ring bowl (Autodesk Fusion 360 design; units mm, degrees)
Autodesk Fusion 360 part; units mm, degrees
note: some values were not read from the file. Set by a fixed rule: which sketch regions a step uses.
sketch "Sketch1" plane through (0, 0, 0) normal (0, 1, 0) x (1, 0, 0) in component "Component"
  circle A0 centre (0, 0) radius 70
  circle A1 centre (0, 0) radius 60
  dimension "d1" = 140
  dimension "d2" = 120
  constraint coincident A0.centre A1.centre
  measures "d1" diameter of A0
  measures "d2" diameter of A1
extrude "Extrude1" add sketch "Sketch1" along normal blind 10 in component "Component"
sketch "Sketch2" plane through (0, 0, 0) normal (0, -1, 0) x (1, 0, 0) in component "Component"
  circle A0 centre (0, 0) radius 60
  circle A1 centre (0, 0) radius 70
  circle A2 centre (0, 0) radius 65
  dimension "d5" = 130
  constraint coincident A0.centre A1.centre
  measures "d5" diameter of A2
extrude "Extrude2" cut sketch "Sketch2" against normal blind 5 contours A2 in component "Component"
fillet "Fillet1" radius 8 1 edges at (-65.2629, 0, 25.3131) in component "Component"
fillet "Fillet2" radius 3 1 edges at (-65.2629, 10, 25.3131) in component "Component"
sketch "Sketch1 (2)" plane through (0, 0, 0) normal (0, 1, 0) x (1, 0, 0)
sketch "Sketch2 (2)" plane through (0, 5, 0) normal (0, -1, 0) x (1, 0, 0)
  circle A0 centre (0, 0) radius 60
  circle A1 centre (0, 0) radius 65
  line L0 (0, 65) -> (0, 60)
  circle A2 centre (0, 65) radius 2.5
  dimension "d12" = 5
  constraint coincident A1 L0.start
  constraint coincident A0 L0.end
  constraint vertical L0
  constraint coincident L0.start A2.centre
  measures "d12" diameter of A2
extrude "Extrude3" add sketch "Sketch2 (2)" along normal blind 5 contours A1 L0 A2 | A1 L0 A2 in component "Component"
sketch "Sketch3" plane through (0, 5, 0) normal (0, -1, 0) x (1, 0, 0)
  arc A0 (-2.4995, 64.9519) -> (2.4995, 64.9519) centre (0, 65) ccw
  arc A1 (-2.4995, 64.9519) -> (2.4995, 64.9519) centre (0, 0) ccw
  circle A2 centre (0, 0) radius 60
  line L0 (0, 0) -> (65, 0)
  line L1 (60, 0) -> (65, 0)
  line L2 (62.5, 0) -> (62.5, 5)
  circle A3 centre (62.5, 0) radius 1.5
  circle A4 centre (62.5, 0) radius 2.5
  dimension "d15" = 3
  constraint coincident A1.centre A2.centre
  constraint coincident A1 L0.end
  constraint horizontal L0
  constraint coincident L0 L1.start
  constraint coincident A2 L1.start
  constraint midpoint L1 L2.start
  constraint perpendicular L0 L2
  constraint coincident L2.start A3.centre
  constraint coincident L1.start A4
  measures "d15" diameter of A3
extrude "Extrude4" cut sketch "Sketch3" against normal blind 8 contours L0 L1 A3 | L0 L1 L2 A3 | L0 L1 L2 A3 in component "Component"
sketch "Sketch4" plane through (0, 10, 0) normal (0, 1, 0) x (-1, 0, 0)
  circle A0 centre (-62.5, 0) radius 1.5
  circle A1 centre (0, 0) radius 60
  spline S0 degree 3 poles (66.9826, -0.0544) (66.9798, -3.5839) (66.6962, -7.1365) (65.4066, -15.147) (64.2177, -19.5741) (60.9452, -28.1855) (58.7925, -32.4438) (54.571, -38.9591) (52.7567, -41.3815) (49.2812, -45.4254) (47.6803, -47.1031) (44.2901, -50.304) (42.5052, -51.8215) (37.7125, -55.4801) (34.5917, -57.4766) (30.1959, -59.8045) (29.0288, -60.3795) (24.6425, -62.3847) (21.2948, -63.6071) (14.4354, -65.5054) (10.9247, -66.1808) (5.8132, -66.749) (4.2232, -66.8682) (-0.9465, -67.0719) (-4.5688, -66.9246) (-11.7531, -66.0427) (-15.3141, -65.3081) (-20.1914, -63.884) (-21.5918, -63.4242) (-27.0293, -61.439) (-30.981, -59.5473) (-38.4414, -55.0269) (-41.9475, -52.3998) (-49.3652, -45.6341) (-53.1424, -41.1806) (-57.8692, -33.8601) (-59.2992, -31.2859) (-61.8945, -25.8003) (-63.0446, -22.8477) (-64.5064, -18.1318) (-64.9652, -16.4118) (-66.4332, -9.8764) (-66.9826, -4.9234) (-66.9826, 0) (-66.9826, 4.32) (-66.5608, 8.6808) (-65.1604, 15.7819) (-64.4214, 18.5676) (-62.6014, 23.9988) (-61.5254, 26.6364) (-58.8362, 32.1852) (-57.1673, 35.0654) (-53.8126, 39.9722) (-52.2034, 42.0514) (-48.7671, 45.9922) (-46.9465, 47.849) (-42.7711, 51.6378) (-40.3816, 53.528) (-34.2083, 57.76) (-30.291, 59.9042) (-21.8991, 63.4774) (-17.3146, 64.8813) (-10.1295, 66.2615) (-7.5969, 66.5989) (-2.5294, 66.9831) (-0.0024, 67.0308) (5.9213, 66.8064) (9.3172, 66.4189) (16.757, 64.9866) (20.7739, 63.8136) (28.6323, 60.7085) (32.533, 58.7137) (39.8722, 53.9991) (43.3082, 51.2809) (49.5367, 45.293) (52.388, 41.9667) (56.5042, 36.0818) (57.974, 33.6687) (60.5889, 28.6976) (61.7315, 26.1491) (63.9224, 20.3074) (64.8858, 16.9825) (66.054, 11.3511) (66.4048, 9.0741) (66.8699, 4.5106) (66.9845, 2.2312) (66.9826, -0.0544) knots -20.91683243 -20.91683243 -20.91683243 -20.91683243 -19.86050435 -19.86050435 -18.50587415 -18.50587415 -17.09682396 -17.09682396 -16.19888273 -16.19888273 -15.5029822 -15.5029822 -14.80708168 -14.80708168 -13.71099921 -13.71099921 -13.32192066 -13.32192066 -12.26415144 -12.26415144 -11.20637725 -11.20637725 -10.72994391 -10.72994391 -9.65424147 -9.65424147 -8.57853406 -8.57853406 -8.13796717 -8.13796717 -6.8419813 -6.8419813 -5.54599042 -5.54599042 -3.83005202 -3.83005202 -2.95401368 -2.95401368 -2.00947943 -2.00947943 -1.47700684 -1.47700684 0 0 0 1.29599087 1.29599087 2.15065358 2.15065358 3.00531628 3.00531628 3.99123717 3.99123717 4.77160343 4.77160343 5.55196968 5.55196968 6.45538036 6.45538036 7.77593024 7.77593024 9.19166653 9.19166653 9.95012483 9.95012483 10.70858313 10.70858313 11.72098027 11.72098027 12.95988373 12.95988373 14.2558746 14.2558746 15.55186047 15.55186047 16.84785135 16.84785135 17.68579426 17.68579426 18.52373718 18.52373718 19.54876425 19.54876425 20.23279834 20.23279834 20.91683243 20.91683243 20.91683243 20.91683243
  circle A2 centre (-62.5, 0) radius 2.5
  constraint concentric A0 A2
extrude "Extrude5" cut sketch "Sketch4" against normal blind 2 contours A2 in component "Component"
sketch "Sketch4 (2)" plane through (0, 10, 0) normal (0, 1, 0) x (-1, 0, 0) in component "Component"
  spline S0 degree 3 poles (66.9826, -0.0544) (66.9798, -3.5839) (66.6962, -7.1365) (65.4066, -15.147) (64.2177, -19.5741) (60.9452, -28.1855) (58.7925, -32.4438) (54.571, -38.9591) (52.7567, -41.3815) (49.2812, -45.4254) (47.6803, -47.1031) (44.2901, -50.304) (42.5052, -51.8215) (37.7125, -55.4801) (34.5917, -57.4766) (30.1959, -59.8045) (29.0288, -60.3795) (24.6425, -62.3847) (21.2948, -63.6071) (14.4354, -65.5054) (10.9247, -66.1808) (5.8132, -66.749) (4.2232, -66.8682) (-0.9465, -67.0719) (-4.5688, -66.9246) (-11.7531, -66.0427) (-15.3141, -65.3081) (-20.1914, -63.884) (-21.5918, -63.4242) (-27.0293, -61.439) (-30.981, -59.5473) (-38.4414, -55.0269) (-41.9475, -52.3998) (-49.3652, -45.6341) (-53.1424, -41.1806) (-57.8692, -33.8601) (-59.2992, -31.2859) (-61.8945, -25.8003) (-63.0446, -22.8477) (-64.5064, -18.1318) (-64.9652, -16.4118) (-66.4332, -9.8764) (-66.9826, -4.9234) (-66.9826, 0) (-66.9826, 4.32) (-66.5608, 8.6808) (-65.1604, 15.7819) (-64.4214, 18.5676) (-62.6014, 23.9988) (-61.5254, 26.6364) (-58.8362, 32.1852) (-57.1673, 35.0654) (-53.8126, 39.9722) (-52.2034, 42.0514) (-48.7671, 45.9922) (-46.9465, 47.849) (-42.7711, 51.6378) (-40.3816, 53.528) (-34.2083, 57.76) (-30.291, 59.9042) (-21.8991, 63.4774) (-17.3146, 64.8813) (-10.1295, 66.2615) (-7.5969, 66.5989) (-2.5294, 66.9831) (-0.0024, 67.0308) (5.9213, 66.8064) (9.3172, 66.4189) (16.757, 64.9866) (20.7739, 63.8136) (28.6323, 60.7085) (32.533, 58.7137) (39.8722, 53.9991) (43.3082, 51.2809) (49.5367, 45.293) (52.388, 41.9667) (56.5042, 36.0818) (57.974, 33.6687) (60.5889, 28.6976) (61.7315, 26.1491) (63.9224, 20.3074) (64.8858, 16.9825) (66.054, 11.3511) (66.4048, 9.0741) (66.8699, 4.5106) (66.9845, 2.2312) (66.9826, -0.0544) knots -20.91683243 -20.91683243 -20.91683243 -20.91683243 -19.86050435 -19.86050435 -18.50587415 -18.50587415 -17.09682396 -17.09682396 -16.19888273 -16.19888273 -15.5029822 -15.5029822 -14.80708168 -14.80708168 -13.71099921 -13.71099921 -13.32192066 -13.32192066 -12.26415144 -12.26415144 -11.20637725 -11.20637725 -10.72994391 -10.72994391 -9.65424147 -9.65424147 -8.57853406 -8.57853406 -8.13796717 -8.13796717 -6.8419813 -6.8419813 -5.54599042 -5.54599042 -3.83005202 -3.83005202 -2.95401368 -2.95401368 -2.00947943 -2.00947943 -1.47700684 -1.47700684 0 0 0 1.29599087 1.29599087 2.15065358 2.15065358 3.00531628 3.00531628 3.99123717 3.99123717 4.77160343 4.77160343 5.55196968 5.55196968 6.45538036 6.45538036 7.77593024 7.77593024 9.19166653 9.19166653 9.95012483 9.95012483 10.70858313 10.70858313 11.72098027 11.72098027 12.95988373 12.95988373 14.2558746 14.2558746 15.55186047 15.55186047 16.84785135 16.84785135 17.68579426 17.68579426 18.52373718 18.52373718 19.54876425 19.54876425 20.23279834 20.23279834 20.91683243 20.91683243 20.91683243 20.91683243
  circle A0 centre (0, 0) radius 60
  circle A1 centre (-62.5, 0) radius 2.5
  circle A2 centre (0, 0) radius 57.5
  dimension "d20" = 115
  constraint coincident A0.centre A2.centre
  measures "d20" diameter of A2
extrude "Extrude6" add sketch "Sketch4 (2)" against normal blind 5 contours A0 in component "Component"
sketch "Sketch5" plane through (0, 10, 0) normal (0, 1, 0) x (-1, 0, 0) in component "Component"
  circle A0 centre (0, 0) radius 57.5
  spline S0 degree 3 poles (66.9826, -0.0544) (66.9798, -3.5839) (66.6962, -7.1365) (65.4066, -15.147) (64.2177, -19.5741) (60.9452, -28.1855) (58.7925, -32.4438) (54.571, -38.9591) (52.7567, -41.3815) (49.2812, -45.4254) (47.6803, -47.1031) (44.2901, -50.304) (42.5052, -51.8215) (37.7125, -55.4801) (34.5917, -57.4766) (30.1959, -59.8045) (29.0288, -60.3795) (24.6425, -62.3847) (21.2948, -63.6071) (14.4354, -65.5054) (10.9247, -66.1808) (5.8132, -66.749) (4.2232, -66.8682) (-0.9465, -67.0719) (-4.5688, -66.9246) (-11.7531, -66.0427) (-15.3141, -65.3081) (-20.1914, -63.884) (-21.5918, -63.4242) (-27.0293, -61.439) (-30.981, -59.5473) (-38.4414, -55.0269) (-41.9475, -52.3998) (-49.3652, -45.6341) (-53.1424, -41.1806) (-57.8692, -33.8601) (-59.2992, -31.2859) (-61.8945, -25.8003) (-63.0446, -22.8477) (-64.5064, -18.1318) (-64.9652, -16.4118) (-66.4332, -9.8764) (-66.9826, -4.9234) (-66.9826, 0) (-66.9826, 4.32) (-66.5608, 8.6808) (-65.1604, 15.7819) (-64.4214, 18.5676) (-62.6014, 23.9988) (-61.5254, 26.6364) (-58.8362, 32.1852) (-57.1673, 35.0654) (-53.8126, 39.9722) (-52.2034, 42.0514) (-48.7671, 45.9922) (-46.9465, 47.849) (-42.7711, 51.6378) (-40.3816, 53.528) (-34.2083, 57.76) (-30.291, 59.9042) (-21.8991, 63.4774) (-17.3146, 64.8813) (-10.1295, 66.2615) (-7.5969, 66.5989) (-2.5294, 66.9831) (-0.0024, 67.0308) (5.9213, 66.8064) (9.3172, 66.4189) (16.757, 64.9866) (20.7739, 63.8136) (28.6323, 60.7085) (32.533, 58.7137) (39.8722, 53.9991) (43.3082, 51.2809) (49.5367, 45.293) (52.388, 41.9667) (56.5042, 36.0818) (57.974, 33.6687) (60.5889, 28.6976) (61.7315, 26.1491) (63.9224, 20.3074) (64.8858, 16.9825) (66.054, 11.3511) (66.4048, 9.0741) (66.8699, 4.5106) (66.9845, 2.2312) (66.9826, -0.0544) knots -20.91683243 -20.91683243 -20.91683243 -20.91683243 -19.86050435 -19.86050435 -18.50587415 -18.50587415 -17.09682396 -17.09682396 -16.19888273 -16.19888273 -15.5029822 -15.5029822 -14.80708168 -14.80708168 -13.71099921 -13.71099921 -13.32192066 -13.32192066 -12.26415144 -12.26415144 -11.20637725 -11.20637725 -10.72994391 -10.72994391 -9.65424147 -9.65424147 -8.57853406 -8.57853406 -8.13796717 -8.13796717 -6.8419813 -6.8419813 -5.54599042 -5.54599042 -3.83005202 -3.83005202 -2.95401368 -2.95401368 -2.00947943 -2.00947943 -1.47700684 -1.47700684 0 0 0 1.29599087 1.29599087 2.15065358 2.15065358 3.00531628 3.00531628 3.99123717 3.99123717 4.77160343 4.77160343 5.55196968 5.55196968 6.45538036 6.45538036 7.77593024 7.77593024 9.19166653 9.19166653 9.95012483 9.95012483 10.70858313 10.70858313 11.72098027 11.72098027 12.95988373 12.95988373 14.2558746 14.2558746 15.55186047 15.55186047 16.84785135 16.84785135 17.68579426 17.68579426 18.52373718 18.52373718 19.54876425 19.54876425 20.23279834 20.23279834 20.91683243 20.91683243 20.91683243 20.91683243
  circle A1 centre (-62.5, 0) radius 2.5
pattern_circular "C-Pattern1" count 3 over 360 about axis through (0, 1.75, 0) along (0, 1, 0) of "Extrude4", "Extrude5" in component "Component"
component "Component" placed x (1, 0, 0) y (0, 1, 0) z (0, 0, 1) at (0, 0, 0)
equation "d48 = ( 13.2 / 2 ) * 1 mm"
equation "d50 = ( 13.2 / 2 ) * 1 mm"
